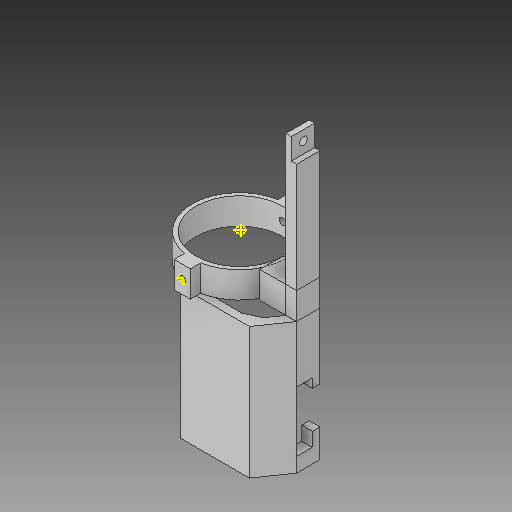
# Autodesk Inventor part: Y-axis-gimbal-part
Saved by Autodesk Inventor 2017 (Build 210142000, 142)
## iProperties
Part Number: Y-axis-gimbal-part
Material: 常规
Document SubType Name: Modeling
Designer: Lenovo
Density: 1 g/cm^3
Appearance: 默认
Sheet Metal Rule: Default
Author: Lenovo
Autodesk Inventor part; units mm, degrees
ref_plane "YZ Plane" through (0, 0, 0) normal (1, 0, 0) x (0, 1, 0)
ref_plane "XZ Plane" through (0, 0, 0) normal (0, 1, 0) x (-1, 0, 0)
ref_plane "XY Plane" through (0, 0, 0) normal (0, 0, 1) x (1, 0, 0)
sketch "Sketch1" plane through (0, 0, 0) normal (0, 1, 0) x (-1, 0, 0)
  circle A0 centre (0, 0) radius 16.5
  circle A1 centre (0, 0) radius 18
  line L0 (3.1, -17.731) -> (3.1, -21.731)
  line L1 (-3.1, -17.731) -> (-3.1, -21.731)
  line L2 (-3.1, -21.731) -> (3.1, -21.731)
  line L3 (3.1, 17.731) -> (3.1, 21.731)
  line L4 (-3.1, 17.731) -> (-3.1, 21.731)
  line L5 (-3.1, 21.731) -> (3.1, 21.731)
  circle A2 centre (0, 0) radius 16.5
  circle A3 centre (0, 0) radius 16.5
  point P0 (-3.1, 19.731)
  dimension "d0" = 33
  dimension "d1" = 36
  dimension "d2" = 4
  dimension "d4" = 4
  dimension "d5" = 4
  dimension "d51" = 33
  dimension "d60" = 33
  constraints: 12 end point, 5 vertical, 4 centre point, 4 coincident, 4 point on circle, 2 perpendicular, 1 midpoint, 1 other
  measures "d0" diameter of A0
  measures "d1" diameter of A1
  measures "d2" distance of L0.start L0.end
  measures "d4" distance of L1.start L1.end
  measures "d5" distance of L3.start L3.end
  measures "d51" diameter of A2
  measures "d60" diameter of A3
extrude "Extrusion1" add sketch "Sketch1" along normal blind 10 contours A0 | A1 | A1 L4 L5 L3 | L0 L2 L1 A1
sketch "Sketch2" plane through (0, 10, 0) normal (0, 1, 0) x (1, 0, 0)
  line L0 (-3.1, -21.731) -> (3.1, -21.731) projected
extrude "Extrusion2" [suppressed]
hole "Hole1" at (0, 5, -21.731) direction (0, 0, 1) diameter 2.621 end through all thread size "M3x0.35" class "6H" standard "ANSI Metric M Profile"
sketch "Sketch3" plane through (0, 0, 0) normal (0, -1, 0) x (1, 0, 0)
  point P0 (0, 0)
hole "Hole2" at (0, 0, 0) direction (0, 1, 0) diameter 33 end through all
sketch "Sketch7" plane through (0, 0, 0) normal (0, -1, 0) x (1, 0, 0)
  circle A0 centre (0, 0) radius 16.5 projected
  line L0 (-3.1, 17.731) -> (-3.1, 21.731) projected
  line L1 (-3.1, 19.4804) -> (23.364, 19.4804)
  line L2 (23.364, 19.4804) -> (30.698, 8.8802)
  line L3 (30.698, 8.8802) -> (30.698, -0.0004)
  line L4 (30.698, -0.0004) -> (26.6263, -0.0004)
  line L5 (26.6263, -0.0004) -> (26.6263, 8.8798)
  line L6 (26.6263, 8.8798) -> (23.1203, 13.9471)
  line L7 (23.1203, 13.9471) -> (17.4825, 16.4996)
  line L8 (17.4825, 16.4996) -> (-0.1192, 16.4996)
  arc A1 (-3.1, 19.4804) -> (-0.1192, 16.4996) centre (-0.1192, 19.4804) ccw
  constraints: 16 end point, 2 parallel, 2 perpendicular, 2 point on circle, 2 tangent, 1 centre point, 1 horizontal, 2 other
extrude "Extrusion4" add sketch "Sketch7" along normal blind 50 contours A1 L1 L2 L3 L4 L5 L6 L7 L8
sketch "Sketch8" plane through (30.698, 0, 8.8802) normal (1, 0, 0) x (0, 0, -1)
  line L0 (8.8806, 0) -> (0, 0) projected
  line L1 (0, 0) -> (0, -50) projected
  line L2 (8.8806, 0) -> (8.8806, -50) projected
  line L3 (8.8806, 0) -> (8.8806, -50) projected
  line L4 (8.8806, -25) -> (5.9549, -25)
  line L5 (5.9549, -25) -> (5.9549, -21.551)
  line L6 (5.9549, -21.551) -> (0.0004, -21.551)
  line L7 (0.0004, 0) -> (0.0004, -50) projected
  line L8 (0.0004, -44.4321) -> (5.9549, -44.4321)
  line L9 (5.9549, -44.4321) -> (5.9549, -39.2166)
  line L10 (5.9549, -39.2166) -> (8.8806, -39.2166)
  point P0 (8.8802, 0)
  constraints: 12 end point, 5 point on line, 4 perpendicular, 1 horizontal, 1 midpoint
extrude "Extrusion5" cut sketch "Sketch8" against normal blind 50 contours L2 L10 L9 L8 L1 L6 L5 L4
sketch "Sketch9" plane through (0, 0, 0) normal (0, 1, 0) x (1, 0, 0)
  line L0 (30.698, 0.0004) -> (30.698, -8.8802) projected
  line L1 (26.6263, -8.8798) -> (26.6263, 0.0004) projected
  line L2 (26.6263, 0.0004) -> (30.698, 0.0004)
  line L3 (30.698, 0.0004) -> (30.698, -8.8802) projected
  line L4 (30.698, -8.8802) -> (26.6263, -8.8798)
  constraints: 4 end point, 1 perpendicular
extrude "Extrusion6" add sketch "Sketch9" along normal blind 60
hole "Hole3" at (30.698, 56.2959, 4.3014) direction (-1, 0, 0) diameter 3 end through all
sketch "Sketch18" plane through (30.698, -50, 8.8802) normal (1, 0, 0) x (0, 0, -1)
  circle A0 centre (4.5788, 106.2959) radius 1.5 projected
  line L0 (0, 50) -> (0, 110) projected
  line L1 (8.8806, 110) -> (0.0004, 110) projected
  line L2 (0, 101.9284) -> (8.8806, 101.9284)
  line L3 (8.8806, 101.9284) -> (8.8806, 110)
  line L4 (8.8806, 110) -> (0, 110)
  line L5 (0, 110) -> (0, 101.9284)
  point P0 (8.8802, 50)
  constraints: 8 end point, 2 parallel, 1 horizontal, 1 perpendicular, 1 point on line
extrude "Extrusion7" cut sketch "Sketch18" against normal blind 2
sketch "Sketch19" plane through (30.698, -50, 8.8802) normal (1, 0, 0) x (0, 0, -1)
  line L0 (8.8806, 101.9284) -> (8.8806, 25) projected
  line L1 (0.0004, 50) -> (0.0004, 28.449) projected
  line L2 (8.8806, 60.2116) -> (0.0004, 60.2116)
  line L3 (0.0004, 60.2116) -> (0.0004, 50)
  line L4 (0.0004, 50) -> (8.8806, 50)
  line L5 (8.8806, 50) -> (8.8806, 60.2116)
  point P0 (8.8802, 50)
  constraints: 8 end point, 2 parallel, 1 horizontal, 1 perpendicular, 1 point on line
extrude "Extrusion8" add sketch "Sketch19" against normal blind 14 separate body
sketch "Sketch21" plane through (0, 10, 0) normal (0, 1, 0) x (1, 0, 0)
  circle A0 centre (0, 0) radius 16.5 projected
  arc A1 (-3.1, 17.731) -> (-3.1, -17.731) centre (0, 0) ccw projected
  circle A2 centre (0, 0) radius 16.5
  dimension "d52" = 33
  constraints: 1 centre point, 1 coincident
  measures "d52" diameter of A2
hole "Hole4" at (0, 10, 0) direction (0, -1, 0) diameter 33 end through all bodies 1
equation "\"BendRadius\" = Thickness"
equation "\"BendReliefWidth\" = Thickness"
equation "\"BendReliefDepth\" = 0.5 * Thickness"
equation "\"CornerReliefSize\" = 4 * Thickness"
equation "\"MinimumRemnant\" = 2 * Thickness"
equation "\"TransitionRadius\" = BendRadius"
equation "\"JacobiRadiusSize\" = Thickness"
equation "\"GapSize\" = Thickness"
equation "\"Thickness\" = 0.5"
body "Solid1"
body "Solid2"
